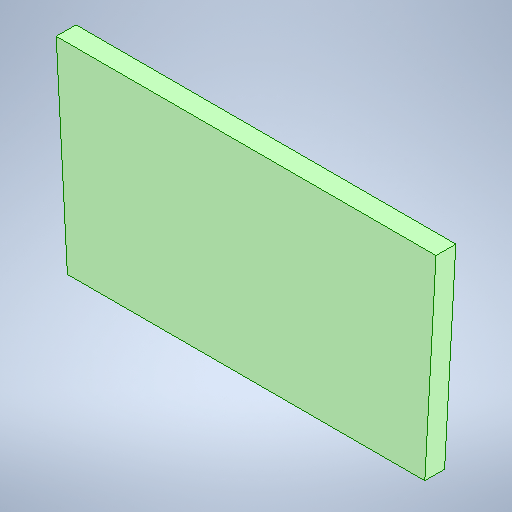
# Autodesk Inventor part: F
Saved by Autodesk Inventor 2025.3 (Build 293356030, 356C)
## iProperties
Created: 2025-07-05
Part Number: F
Material: Generic
Document SubType Name: Modeling
Designer: steve
Density: 1 g/cm^3
Appearance: Default(1)
Author: steve
Autodesk Inventor part; units mm, degrees
ref_plane "YZ Plane" through (0, 0, 0) normal (1, 0, 0) x (0, 1, 0)
ref_plane "XZ Plane" through (0, 0, 0) normal (0, 1, 0) x (-1, 0, 0)
ref_plane "XY Plane" through (0, 0, 0) normal (0, 0, 1) x (1, 0, 0)
sketch "Sketch1" plane through (0, 0, 0) normal (0, 0, 1) x (1, 0, 0)
  line L0 (-27.055, 0) -> (27.055, 0)
  line L1 (-28.75, 30.37) -> (28.75, 30.37)
  line L2 (27.055, 0) -> (28.75, 30.37)
  line L3 (-28.75, 30.37) -> (-27.055, 0)
  line L4 (0, 30.37) -> (0, 16.4508)
  point P0 (0, 0)
  point P1 (0, 0)
  dimension "d0" = 54.11
  dimension "d1" = 57.5
  dimension "d2" = 30.37
  dimension "d3" = 0
  constraints: 10 end point, 2 horizontal, 2 midpoint, 1 coincident, 1 vertical
  measures "d0" distance of L0.start L0.end
  measures "d1" distance of L1.start L1.end
  measures "d2" distance between parallel lines of L1 L0
  measures "d3" horizontal distance of point (0, 0) L4.start
extrude "Extrusion1" add sketch "Sketch1" along normal blind 3
body "Solid1"
